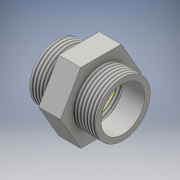
# Autodesk Inventor part: niple 4 inch
Saved by Autodesk Inventor 2016 (Build 200138000, 138)
## iProperties
Created: 2019-01-23
Part Number: niple 4 inch
Material: Generic
Document SubType Name: Modeling
Designer: Cliente
Density: 1 g/cm^3
Appearance: Default
Author: Cliente
Autodesk Inventor part; units mm, degrees
ref_plane "YZ Plane" through (0, 0, 0) normal (1, 0, 0) x (0, 1, 0)
ref_plane "XZ Plane" through (0, 0, 0) normal (0, 1, 0) x (-1, 0, 0)
ref_plane "XY Plane" through (0, 0, 0) normal (0, 0, 1) x (1, 0, 0)
sketch "Sketch1" plane through (0, 0, 0) normal (1, 0, 0) x (0, 1, 0)
  circle A0 centre (0, 0) radius 50
  line L0 (-36.9504, -64) -> (-73.9008, 0)
  line L1 (-73.9008, 0) -> (-36.9504, 64)
  line L2 (-36.9504, 64) -> (36.9504, 64)
  line L3 (36.9504, 64) -> (73.9008, 0)
  line L4 (73.9008, 0) -> (36.9504, -64)
  line L5 (36.9504, -64) -> (-36.9504, -64)
  dimension "d0" = 100
  dimension "d1" = 64
  constraints: 12 end point, 2 coincident, 1 centre point, 13 other
  measures "d0" diameter of A0
  measures "d1" distance from line of L5 point (0, 0)
extrude "Extrusion1" add sketch "Sketch1" along normal mid plane 40
sketch "Sketch3" plane through (0, 0, 0) normal (1, 0, 0) x (0, 1, 0)
  circle A0 centre (0, 0) radius 50 projected
  constraints: 1 coincident
thread "Thread1" size "M100x6" class "6H" standard "ANSI Metric M Profile" full length
sketch "Sketch4" plane through (20, 0, 0) normal (1, 0, 0) x (0, 0, -1)
  circle A0 centre (0, 0) radius 50 projected
  circle A1 centre (0, 0) radius 40
  dimension "d12" = 10
  constraints: 1 centre point
  measures "d12" radial gap between concentric circles of A0 A1
extrude "Extrusion4" add sketch "Sketch4" along normal blind 40
thread "Thread2" size "M100x6" class "6g" standard "ANSI Metric M Profile" full length
mirror "Mirror1" about plane through (0, 0, 0) normal (1, 0, 0) of "Extrusion4"
thread "Thread3" size "M100x6" class "6g" standard "ANSI Metric M Profile" full length
body "Solid1"
